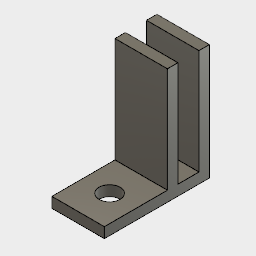
ultrasonic_mount (Autodesk Fusion 360 design; units mm, degrees)
Autodesk Fusion 360 part; units mm, degrees
sketch "Sketch1" plane through (0, 0, 0) normal (0, 1, 0) x (1, 0, 0)
  line L0 (0, 0) -> (5, 0)
  line L1 (5, 0) -> (5, -10)
  line L2 (5, -10) -> (0, -10)
  line L3 (0, -10) -> (0, 0)
  line L4 (0, -1) -> (5, -1)
  line L5 (0, -3) -> (5, -3)
  line L6 (0, -4) -> (5, -4)
  circle A0 centre (2.5, -7) radius 1
  dimension "d1" = 10
  dimension "d2" = 5
  dimension "d3" = 2
  dimension "d4" = 1
  dimension "d5" = 1
  dimension "d6" = 2
  measures "d1" distance of L0.end L1.end
  measures "d2" distance of L0.start L0.end
  measures "d3" distance of L4.start L5.start
  measures "d4" distance of L0.start L4.start
  measures "d5" distance of L5.start L6.start
  measures "d6" diameter of A0
ref_plane "WorkPlane1" through (2.5, 5, 3.5) normal (0, 1, 0) x (1, 0, 0)
ref_plane "WorkPlane2" through (2.5, 5, 0.5) normal (0, 1, 0) x (1, 0, 0)
ref_plane "WorkPlane3" through (2.5, 1, 2) normal (0, 1, 0) x (1, 0, 0)
ref_plane "WorkPlane4" through (2.5, 1, 7) normal (0, 1, 0) x (1, 0, 0)
sketch "Sketch2" plane through (0, 0, 0) normal (1, 0, 0) x (0, 0, -1)
  line L0 (-1, 11) -> (-1, 1)
  line L1 (-1, 1) -> (-3, 1)
  line L2 (-3, 1) -> (-3, 11)
  line L3 (-3, 11) -> (-4, 11)
  line L4 (-4, 11) -> (-4, 1)
  line L5 (-4, 1) -> (-10, 1)
  line L6 (-10, 1) -> (-10, 0)
  line L7 (-10, 0) -> (0, 0)
  line L8 (0, 11) -> (-1, 11)
  line L9 (0, 0) -> (-10, 0)
  line L10 (0, 11) -> (0, 1)
  line L11 (0, 1) -> (0, 0)
  line L12 (0, 1) -> (0, 11)
  point P0 (-10, 0)
  dimension "d11" = 10
  dimension "d12" = 2
  dimension "d13" = 10
  dimension "d14" = 1
  dimension "d15" = 1
  dimension "d17" = 6
  dimension "d18" = 1
  dimension "d20" = 1
  dimension "d21" = 10
  measures "d11" distance of L3.end L4.end
  measures "d12" distance of L0.end L1.end
  measures "d13" distance of L7.end P0
  measures "d14" distance of L2.end L3.end
  measures "d15" distance of L0.start L8.start
  measures "d17" distance of L4.end L5.end
  measures "d18" distance of L5.end P0
  measures "d20" distance of L7.end L10.end
  measures "d21" distance of L8.start L10.end
extrude "Extrude1" add sketch "Sketch2" along normal blind 5
extrude "Extrude2" cut sketch "Sketch1" along normal blind 1 contours A0
named bodies: "ultrasonic_mount"
